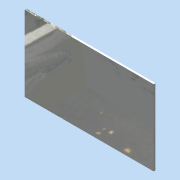
# Autodesk Inventor part: FacePlate
Saved by Autodesk Inventor 2011 SP1 (Build 150282100, 282)
## iProperties
Created: 2011-08-14
Part Number: FacePlate
Document SubType Name: Modeling
Designer: dgitz
Density: 1 g/cm^3
Author: dgitz
Autodesk Inventor part; units mm, degrees
ref_plane "YZ Plane" through (0, 0, 0) normal (1, 0, 0) x (0, 1, 0)
ref_plane "XZ Plane" through (0, 0, 0) normal (0, 1, 0) x (-1, 0, 0)
ref_plane "XY Plane" through (0, 0, 0) normal (0, 0, 1) x (1, 0, 0)
sketch "Sketch1" plane through (0, 0, 0) normal (0, 0, 1) x (1, 0, 0)
  line L0 (-18.3787, 42.1897) -> (68.4893, 42.1897)
  line L1 (68.4893, 42.1897) -> (68.4893, -8.6103)
  line L2 (68.4893, -8.6103) -> (-18.3787, -8.6103)
  line L3 (-18.3787, -8.6103) -> (-18.3787, 42.1897)
  point P0 (0, 0)
  dimension "d0" = 86.868
  dimension "d1" = 50.8
  constraints: 8 end point, 2 parallel, 1 horizontal, 1 perpendicular
  measures "d0" distance between parallel lines of L1 L3
  measures "d1" distance between parallel lines of L2 L0
extrude "Extrusion1" add sketch "Sketch1" along normal blind 1.27
body "Solid1"
